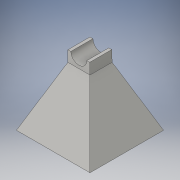
# Autodesk Inventor part: SupportForMouseWire
Saved by Autodesk Inventor 2016 (Build 200138000, 138)
## iProperties
Created: 2015-07-27
Part Number: SupportForMouseWire
Material: Generic
Document SubType Name: Modeling
Designer: steele
Density: 1 g/cm^3
Appearance: Default
Author: steele
Autodesk Inventor part; units mm, degrees
ref_plane "YZ Plane" through (0, 0, 0) normal (1, 0, 0) x (0, 1, 0)
ref_plane "XY Plane" through (0, 0, 0) normal (0, 0, 1) x (1, 0, 0)
sketch "Sketch1" plane through (0, 0, 0) normal (0, 1, 0) x (-1, 0, 0)
  line L0 (-15.875, 15.875) -> (-15.875, -15.875)
  line L1 (-15.875, -15.875) -> (15.875, -15.875)
  line L2 (15.875, -15.875) -> (15.875, 15.875)
  line L3 (15.875, 15.875) -> (-15.875, 15.875)
  line L4 (-15.875, 15.875) -> (15.875, -15.875) construction
  line L5 (-15.875, -15.875) -> (15.875, 15.875) construction
  point P0 (0, 0)
  dimension "base" = 31.75
  constraints: 12 end point, 2 midpoint, 2 parallel, 2 perpendicular, 1 vertical
  measures "base" distance of L2.end L0.start
ref_plane "Work Plane1" through (0, 25.4, 0) normal (0, 1, 0) x (-1, 0, 0)
sketch "Sketch2" plane through (0, 25.4, 0) normal (0, 1, 0) x (-1, 0, 0)
  line L0 (-4.7625, 4.7625) -> (-4.7625, -4.7625)
  line L1 (-4.7625, -4.7625) -> (4.7625, -4.7625)
  line L2 (4.7625, -4.7625) -> (4.7625, 4.7625)
  line L3 (4.7625, 4.7625) -> (-4.7625, 4.7625)
  line L4 (-4.7625, 4.7625) -> (4.7625, -4.7625) construction
  line L5 (-4.7625, -4.7625) -> (4.7625, 4.7625) construction
  point P0 (0, 0)
  dimension "topOfPyramid" = 9.525
  constraints: 12 end point, 2 midpoint, 2 parallel, 2 perpendicular, 1 vertical
  measures "topOfPyramid" distance of L2.end L0.start
loft "Loft1" add profiles "Sketch1", "Sketch2"
sketch "Sketch3" plane through (0, 0, 0) normal (0, 0, 1) x (1, 0, 0)
  arc A0 (-3.4925, 30.099) -> (3.3655, 30.099) centre (-0.0635, 30.099) ccw
  arc A1 (-4.7625, 30.099) -> (4.6355, 30.099) centre (-0.0635, 30.099) ccw
  line L0 (4.7625, 25.4) -> (-4.7625, 25.4) projected
  line L1 (3.3655, 30.099) -> (4.6355, 30.099)
  line L2 (-3.4925, 30.099) -> (-4.7625, 30.099)
  line L3 (-4.7625, 30.099) -> (-4.7625, 25.4)
  line L4 (4.6355, 30.099) -> (4.7625, 25.4)
  line L5 (15.875, 0) -> (4.7625, 25.4) projected
  line L6 (4.7625, 25.4) -> (0, 25.4)
  line L7 (-4.7625, 25.4) -> (4.7625, 25.4) projected
  line L8 (-4.7625, 25.4) -> (0, 25.4)
  point P0 (0, 0)
  dimension "innerDiamForRope" = 6.858
  dimension "centerForRope" = 4.699
  dimension "outsideDiam" = 9.398
  constraints: 12 end point, 4 point on circle, 2 centre point, 1 coincident, 1 collinear, 1 horizontal, 1 midpoint, 1 perpendicular, 1 point on line, 1 tangent
  measures "innerDiamForRope" diameter of A0
  measures "centerForRope" distance from line of L0 A0.centre
  measures "outsideDiam" diameter of A1
extrude "Extrusion1" add sketch "Sketch3" along normal mid plane 9.525
equation "\"centerForRope\" = 0.5 * outsideDiam"
equation "\"widthOfTop\" = topOfPyramid"
body "Solid1"
